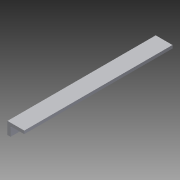
# Autodesk Inventor part: Y_shaft_support_cross_bar
Saved by Autodesk Inventor 2013 (Build 170138000, 138)
## iProperties
Created: 2013-09-23
Part Number: Y_shaft_support_cross_bar
Material: Aluminum 6061
Document SubType Name: Modeling
Designer: Ian
Density: 2.71 g/cm^3
Mass: 288.336 g
Surface Area: 374.879 cm^2
Volume: 106.397 cm^3
d0: 1.000 in
d1: 1.375 in
d2: 0.250 in
d3: 0.250 in
d4: 0.125 in
d5: 12.145 in
d6: 0.00 deg
Author: Ian
Autodesk Inventor part; units mm, degrees
ref_plane "YZ Plane" through (0, 0, 0) normal (1, 0, 0) x (0, 1, 0)
ref_plane "XZ Plane" through (0, 0, 0) normal (0, 1, 0) x (-1, 0, 0)
ref_plane "XY Plane" through (0, 0, 0) normal (0, 0, 1) x (1, 0, 0)
sketch "Sketch1" plane through (0, 0, 0) normal (0, 0, 1) x (1, 0, 0)
  line L0 (0, 0) -> (0, -25.4)
  line L1 (0, 0) -> (34.925, 0)
  line L2 (0, -25.4) -> (6.35, -25.4)
  line L3 (34.925, 0) -> (34.925, -6.35)
  line L4 (34.925, -6.35) -> (9.525, -6.35)
  line L5 (6.35, -9.525) -> (6.35, -25.4)
  arc A0 (9.525, -6.35) -> (6.35, -9.525) centre (9.525, -9.525) ccw
  dimension "d0" = 25.4
  dimension "d1" = 34.925
  dimension "d2" = 6.35
  dimension "d3" = 6.35
  dimension "d4" = 3.175
  constraints: 12 end point, 3 perpendicular, 2 parallel, 2 point on circle, 2 tangent, 1 centre point, 1 vertical
  measures "d0" distance of L0.start L0.end
  measures "d1" distance of L0.start L1.end
  measures "d2" distance of L0.end L2.end
  measures "d3" distance of L1.end L3.end
  measures "d4" radius of A0
extrude "Extrusion1" add sketch "Sketch1" along normal blind 308.483
equation "\"d2\" = d3"
body "Solid1"
